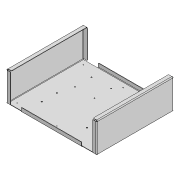
# Autodesk Inventor part: Controller_A
Saved by Autodesk Inventor 2020 (Build 240168000, 168)
## iProperties
Created: 2021-08-23
Part Number: Controller_A
Material: 一般
Document SubType Name: Sheet Metal
Designer: magnarecta
Density: 1 g/cm^3
Sheet Metal Rule: Default_mm
Appearance: 既定
Author: magnarecta
Autodesk Inventor part; units mm, degrees
ref_plane "YZ Plane" through (0, 0, 0) normal (1, 0, 0) x (0, 1, 0)
ref_plane "XZ Plane" through (0, 0, 0) normal (0, 1, 0) x (-1, 0, 0)
ref_plane "XY Plane" through (0, 0, 0) normal (0, 0, 1) x (1, 0, 0)
sketch "スケッチ1" plane through (0, 0, 0) normal (0, 1, 0) x (-1, 0, 0)
  line L0 (-150, -125) -> (150, -125)
  line L1 (150, -125) -> (150, 125)
  line L2 (150, 125) -> (-150, 125)
  line L3 (-150, 125) -> (-150, -125)
  line L4 (-150, -125) -> (150, 125) construction
  line L5 (150, -125) -> (-150, 125) construction
  point P0 (0, 0)
  dimension "d0" = 300
  dimension "d1" = 250
  measures "d0" distance of L1.end L2.end
  measures "d1" distance of L2.end L0.start
extrude "プレート1" add sketch "スケッチ1" along normal blind 1.5
sketch "スケッチ2" plane through (0, 1.5, 0) normal (0, 1, 0) x (1, 0, 0)
  line L0 (55, -65) -> (-95, -65)
  line L1 (-95, -65) -> (-95, -15)
  line L2 (-95, -15) -> (55, -15)
  line L3 (55, -15) -> (55, -65)
  line L4 (55, -65) -> (-95, -15) construction
  line L5 (-95, -65) -> (55, -15) construction
  point P0 (0, 0)
  point P1 (-20, -40)
  dimension "d3" = 150
  dimension "d4" = 50
  dimension "d118" = 40
  dimension "d119" = 20
  constraints: 12 end point, 2 midpoint, 2 parallel, 1 horizontal, 1 perpendicular
  measures "d3" distance of L0.start L0.end
  measures "d4" distance of L2.end L0.start
  measures "d118" vertical distance of point (-20, -40) point (0, 0)
  measures "d119" horizontal distance of point (-20, -40) point (0, 0)
hole "穴1" at (55, 1.5, 65) at (55, 1.5, 15) at (-95, 1.5, 15) at (-95, 1.5, 65) direction (0, -1, 0) diameter 4.2 end through all
sketch "スケッチ3" plane through (148.5, 0, -125) normal (1, 0, 0) x (0, 1, 0)
  line L0 (0, 250) -> (0, 0)
  line L1 (0, 0) -> (100, 0)
  line L2 (100, 0) -> (100, 250)
  line L3 (100, 250) -> (0, 250)
  constraints: 6 end point, 1 horizontal, 1 perpendicular, 1 vertical
edge flange "フランジ1" height 100 angle 90 thickness 1.5 bend radius 1.5 thickness toward (1, 0, 0) relief straight relief width 1.5 relief depth 0.75 corner gap 1.5 corner form 0 edges at (150, 1.5, 0) (-150, 1.5, 0) wall of the first edge with corners at (148.5, 0, 125) (148.5, 0, -125) (148.5, 100, -125) (148.5, 100, 125)
bend "曲げ1"
corner "コーナー1"
sketch "スケッチ5" plane through (0, 1.5, 0) normal (0, 1, 0) x (1, 0, 0)
  line L0 (-17.5, 32.5) -> (-82.5, 32.5)
  line L1 (-82.5, 32.5) -> (-82.5, 87.5)
  line L2 (-82.5, 87.5) -> (-17.5, 87.5)
  line L3 (-17.5, 87.5) -> (-17.5, 32.5)
  line L4 (-17.5, 32.5) -> (-82.5, 87.5) construction
  line L5 (-82.5, 32.5) -> (-17.5, 87.5) construction
  point P0 (0, 0)
  point P1 (-50, 60)
  dimension "d34" = 65
  dimension "d35" = 55
  dimension "d36" = 60
  dimension "d37" = 50
  constraints: 12 end point, 2 midpoint, 2 parallel, 1 horizontal, 1 perpendicular
  measures "d34" distance of L1.end L2.end
  measures "d35" distance of L2.end L0.start
  measures "d36" vertical distance of point (-50, 60) point (0, 0)
  measures "d37" horizontal distance of point (-50, 60) point (0, 0)
hole "穴2" at (-82.5, 1.5, -32.5) at (-17.5, 1.5, -87.5) at (-82.5, 1.5, -87.5) at (-17.5, 1.5, -32.5) direction (0, -1, 0) diameter 3.242 end through all thread size "M4x0.7" class "6H" standard "ISO Metric profile"
sketch "スケッチ10" plane through (-150, 98.5, 125) normal (0, 1, 0) x (-1, 0, 0)
  line L0 (0, -250) -> (0, 0)
  line L1 (0, 0) -> (-14, 0)
  line L2 (-14, 0) -> (-14, -250)
  line L3 (-14, -250) -> (0, -250)
  constraints: 6 end point, 1 horizontal, 1 perpendicular, 1 vertical
edge flange "フランジ6" height 14 angle 90 thickness 1.5 bend radius 1.5 thickness toward (0, 1, 0) relief straight relief width 1.5 relief depth 0.75 corner gap 1.5 corner form 0 edges at (-148.5, 100, 0) (148.5, 100, 0) wall of the first edge with corners at (-150, 98.5, -125) (-150, 98.5, 125) (-136, 98.5, 125) (-136, 98.5, -125)
bend "曲げ6"
corner "コーナー6"
sketch "スケッチ11" plane through (-147, 3, 126.5) normal (0, 0, 1) x (1, 0, 0)
  line L0 (0, 94) -> (0, 0)
  line L1 (0, 0) -> (11, 0)
  line L2 (11, 0) -> (11, 94)
  line L3 (11, 94) -> (0, 94)
  constraints: 6 end point, 1 horizontal, 1 perpendicular, 1 vertical
edge flange "フランジ7" height 14 angle 90 thickness 1.5 bend radius 1.5 thickness toward (0, 0, 1) relief straight relief width 1.5 relief depth 0.75 corner gap 1.5 corner form 0 edges at (-148.5, 50, 125) (-148.5, 50, -125) (148.5, 50, 125) (148.5, 50, -125) wall of the first edge with corners at (-147, 97, 126.5) (-147, 3, 126.5) (-136, 3, 126.5) (-136, 97, 126.5)
bend "曲げ7"
corner "コーナー7"
sketch "スケッチ12" plane through (0, 0, 0) normal (0, -1, 0) x (1, 0, 0)
  circle A0 centre (-82.5, -87.5) radius 1.621 projected
  circle A1 centre (-82.5, -32.5) radius 1.621 projected
  circle A2 centre (-17.5, -87.5) radius 1.621 projected
  circle A3 centre (-17.5, -32.5) radius 1.621 projected
  circle A4 centre (-95, 15) radius 2.1 projected
  circle A5 centre (55, 65) radius 2.1 projected
  circle A6 centre (55, 15) radius 2.1 projected
  circle A7 centre (-95, 65) radius 2.1 projected
  line L0 (-147, 125) -> (-147, -125) projected
  line L1 (147, -125) -> (-147, -125) projected
  line L2 (147, -125) -> (147, 125) projected
  line L3 (-147, 125) -> (147, 125) projected
  line L4 (-100, 127) -> (100, 127)
  line L5 (100, 127) -> (100, -127)
  line L6 (100, -127) -> (-100, -127)
  line L7 (-100, -127) -> (-100, 127)
  point P0 (0, 0)
  point P1 (-100, 125)
  point P2 (100, 125)
  point P3 (100, -125)
  point P4 (-100, -125)
  dimension "d101" = 2
  dimension "d102" = 2
  dimension "d103" = 100
  dimension "d104" = 200
  constraints: 8 end point, 2 parallel, 1 horizontal, 1 perpendicular
  measures "d101" distance between parallel lines of L1 L6
  measures "d102" distance between parallel lines of L4 L3
  measures "d103" distance from line of point (0, 0) L7
  measures "d104" distance of L4.start L4.end
extrude "押し出し2" add sketch "スケッチ12" against normal up to surface (1.5 mm away) contours L7 L4 L5 L3 | L1 L5 L6 L7
sketch "スケッチ13" plane through (100, 1.5, 127) normal (0, 0, 1) x (1, 0, 0)
  line L0 (-200, 0) -> (0, 0)
  line L1 (0, 0) -> (0, 12.5)
  line L2 (0, 12.5) -> (-200, 12.5)
  line L3 (-200, 12.5) -> (-200, 0)
  constraints: 6 end point, 1 horizontal, 1 perpendicular, 1 vertical
edge flange "フランジ8" height 14 angle 90 thickness 1.5 bend radius 1.5 thickness toward (0, 0, 1) relief straight relief width 1.5 relief depth 0.75 corner gap 1.5 corner form 0 edges at (0, 1.5, 127) (0, 1.5, -127) wall of the first edge with corners at (-100, 1.5, 127) (100, 1.5, 127) (100, 14, 127) (-100, 14, 127)
bend "曲げ8"
corner "コーナー8"
fillet "フィレット2" radius 2 16 edges at (-136, 3, 127.25) (-100, 14, 127.75) (-136, 97, 127.25) (-136, 99.25, 125) (-136, 97, -127.25) (-136, 99.25, -125) (-100, 14, -127.75) (-136, 3, -127.25) (100, 14, -127.75) (136, 3, -127.25) (136, 97, -127.25) (136, 99.25, -125) (136, 99.25, 125) (136, 97, 127.25) (100, 14, 127.75) (136, 3, 127.25)
sketch "スケッチ14" plane through (0, 0, 0) normal (0, -1, 0) x (1, 0, 0)
  line L0 (-132, -110) -> (132, -110)
  line L1 (132, -110) -> (132, 110)
  line L2 (132, 110) -> (-132, 110)
  line L3 (-132, 110) -> (-132, -110)
  line L4 (-132, -110) -> (132, 110) construction
  line L5 (132, -110) -> (-132, 110) construction
  line L6 (100, 125) -> (147, 125) projected
  line L7 (147, -125) -> (147, 125) projected
  point P0 (0, 0)
  point P1 (0, 110)
  point P2 (0, -110)
  dimension "d120" = 15
  dimension "d121" = 15
  constraints: 12 end point, 4 midpoint, 2 parallel, 1 horizontal, 1 perpendicular
  measures "d120" distance between parallel lines of L2 L6
  measures "d121" distance between parallel lines of L7 L1
hole "穴3" at (0, 0, 110) at (0, 0, -110) at (132, 0, 110) at (132, 0, -110) at (-132, 0, 110) at (-132, 0, -110) direction (0, 1, 0) diameter 2.459 end through all thread size "M3x0.5" class "6H" standard "ISO Metric profile"
equation "\"d12\" = Thickness"
equation "\"d2\" = Thickness"
equation "\"d14\" = BendReliefWidth"
equation "\"d15\" = BendReliefDepth"
equation "\"d16\" = MinimumRemnant"
equation "\"d17\" = TransitionRadius"
equation "\"d20\" = BendRadius"
equation "\"d21\" = CornerReliefSize"
equation "\"d22\" = GapSize"
equation "\"d23\" = JacobiRadiusSize"
equation "\"d81\" = BendReliefWidth"
equation "\"d82\" = BendReliefDepth"
equation "\"d83\" = MinimumRemnant"
equation "\"d84\" = TransitionRadius"
equation "\"d87\" = BendRadius"
equation "\"d88\" = CornerReliefSize"
equation "\"d89\" = GapSize"
equation "\"d90\" = JacobiRadiusSize"
equation "\"d91\" = BendReliefWidth"
equation "\"d92\" = BendReliefDepth"
equation "\"d93\" = MinimumRemnant"
equation "\"d94\" = TransitionRadius"
equation "\"d97\" = BendRadius"
equation "\"d98\" = CornerReliefSize"
equation "\"d99\" = GapSize"
equation "\"d100\" = JacobiRadiusSize"
equation "\"d107\" = BendReliefWidth"
equation "\"d108\" = BendReliefDepth"
equation "\"d109\" = MinimumRemnant"
equation "\"d110\" = TransitionRadius"
equation "\"d113\" = BendRadius"
equation "\"d114\" = CornerReliefSize"
equation "\"d115\" = GapSize"
equation "\"d116\" = JacobiRadiusSize"
equation "\"BendRadius\" = Thickness"
equation "\"BendReliefWidth\" = Thickness"
equation "\"BendReliefDepth\" = 0.5 * Thickness"
equation "\"CornerReliefSize\" = 4 * Thickness"
equation "\"MinimumRemnant\" = 2 * Thickness"
equation "\"TransitionRadius\" = BendRadius"
equation "\"JacobiRadiusSize\" = BendRadius"
equation "\"GapSize\" = Thickness"
equation "\"Thickness\" = 1.5"
